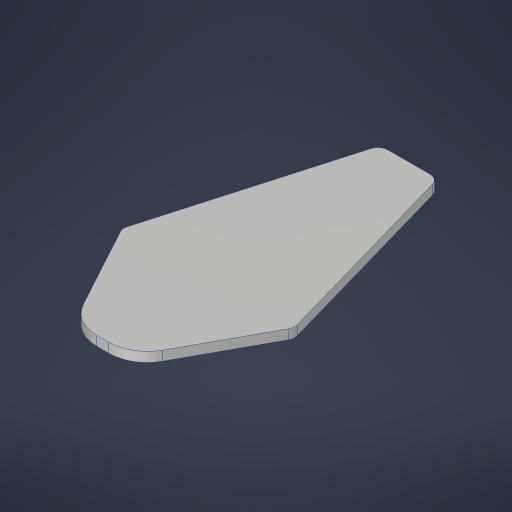
# Autodesk Inventor part: CL4-003
Saved by Autodesk Inventor 2023.4 (Build 274418000, 418)
## iProperties
Created: 2025-02-03
Part Number: CL4-003
Material: Aluminum 6061
Document SubType Name: Modeling
Designer: brand
Density: 2.7 g/cm^3
Appearance: Aluminum - Flat
Author: brand
Autodesk Inventor part; units mm, degrees
ref_plane "YZ Plane" through (0, 0, 0) normal (1, 0, 0) x (0, 1, 0)
ref_plane "XZ Plane" through (0, 0, 0) normal (0, 1, 0) x (-1, 0, 0)
ref_plane "XY Plane" through (0, 0, 0) normal (0, 0, 1) x (1, 0, 0)
sketch "Sketch1" plane through (0, 0, 0) normal (0, 1, 0) x (-1, 0, 0)
  line L0 (19.05, -203.2) -> (-19.05, -203.2)
  line L1 (-19.05, -203.2) -> (-57.15, -69.85)
  line L2 (19.05, -203.2) -> (57.15, -69.85)
  line L3 (57.15, -69.85) -> (19.05, 0)
  line L4 (19.05, 0) -> (-19.05, 0)
  line L5 (-19.05, 0) -> (-57.15, -69.85)
  line L6 (57.15, -69.85) -> (-57.15, -69.85) construction
  line L7 (-12.7, -50.8) -> (12.7, -50.8) construction
  line L8 (12.7, -50.8) -> (12.7, 0) construction
  line L9 (12.7, 0) -> (-12.7, 0) construction
  line L10 (-12.7, 0) -> (-12.7, -50.8) construction
  point P0 (0, 0)
  point P1 (0, -203.2)
  point P2 (0, -69.85)
  point P3 (0, 0)
  dimension "d0" = 25.4
  dimension "d1" = 50.8
  dimension "d2" = 6.35
  dimension "d3" = 114.3
  dimension "d4" = 203.2
  dimension "d5" = 19.05
  dimension "d6" = 38.1
  constraints: 22 end point, 4 horizontal, 4 midpoint, 2 coincident, 2 parallel, 2 vertical alignment, 1 horizontal alignment, 1 perpendicular
  measures "d0" distance of L7.start L7.end
  measures "d1" distance of L7.end L8.end
  measures "d2" distance of L4.end L9.end
  measures "d3" distance of L2.end L1.end
  measures "d4" distance from line of L8.end L0
  measures "d5" distance between parallel lines of L7 L6
  measures "d6" distance of L0.start L0.end
extrude "Extrusion1" add sketch "Sketch1" along normal mid plane 6.35
fillet "Fillet1" radius 6.604 4 edges at (57.15, 0, -69.85) (19.05, 0, -203.2) (-19.05, 0, -203.2) (-57.15, 0, -69.85)
fillet "Fillet2" radius 25.4 2 edges at (-19.05, 0, 0) (19.05, 0, 0)
body "Solid1"
